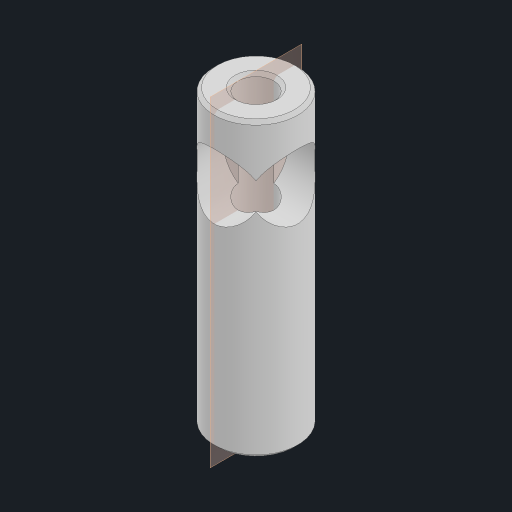
# Autodesk Inventor part: motor_shaft_adapter
Saved by Autodesk Inventor 2023 (Build 270158000, 158)
## iProperties
Created: 2024-04-12
Part Number: motor_shaft_adapter
Material: Generic
Document SubType Name: Modeling
Designer: szymo
Density: 1 g/cm^3
Appearance: Default
Author: szymo
Autodesk Inventor part; units mm, degrees
ref_plane "XZ Plane" through (0, 0, 0) normal (0, 1, 0) x (-1, 0, 0)
ref_plane "XY Plane" through (0, 0, 0) normal (0, 0, 1) x (1, 0, 0)
sketch "Sketch1" plane through (0, 0, 0) normal (0, 1, 0) x (-1, 0, 0)
  circle A0 centre (0, 0) radius 1.1
  circle A1 centre (0, 0) radius 2.575
  dimension "d0" = 2.2
  dimension "d1" = 5.15
  constraints: 2 centre point, 2 coincident
  measures "d0" diameter of A0
  measures "d1" diameter of A1
extrude "Extrusion1" add sketch "Sketch1" along normal blind 18
sketch "Sketch2" plane through (0, 0, 0) normal (0, 0, 1) x (1, 0, 0)
  line L0 (2.575, 18) -> (-2.575, 18) projected
  line L1 (2.575, 0) -> (-2.575, 0) projected
  line L2 (-2.575, 0) -> (-2.575, 18) projected
  line L3 (-2.575, 16) -> (2.5173, 16)
  line L4 (2.575, 18) -> (-2.575, 18) projected
  line L5 (0, 18) -> (0, 0)
  circle A0 centre (0, 14) radius 2
  dimension "d4" = 2
  dimension "d5" = 4
  constraints: 4 end point, 2 point on line, 1 centre point, 1 horizontal, 1 midpoint, 1 parallel, 1 tangent, 1 vertical
  measures "d4" distance between parallel lines of L0 L3
  measures "d5" diameter of A0
extrude "Extrusion2" cut sketch "Sketch2" along normal blind 12 contours A0 L5 | L5 A0
sketch "Sketch3" plane through (0, 0, 0) normal (1, 0, 0) x (0, 1, 0)
  line L0 (18, -2.575) -> (18, 2.575) projected
  line L1 (0, -2.575) -> (0, 2.575) projected
  line L2 (0, 2.575) -> (18, 2.575) projected
  line L3 (16, 2.575) -> (16, -2.525)
  line L4 (18, 1.1) -> (18, -1.1) projected
  line L5 (18, 0) -> (0, 0)
  circle A0 centre (14, 0) radius 2
  point P0 (14, 1.6219)
  dimension "d8" = 2
  dimension "d9" = 4
  constraints: 4 end point, 2 point on line, 1 centre point, 1 horizontal, 1 midpoint, 1 parallel, 1 perpendicular, 1 tangent
  measures "d8" distance between parallel lines of L0 L3
  measures "d9" diameter of A0
extrude "Extrusion3" cut sketch "Sketch3" along normal up to next contours A0 L5 | L5 A0
chamfer "Chamfer1" distance 0.2 angle 45 4 edges at (1.1, 0, 0) (2.575, 0, 0) (1.1, 18, 0) (2.575, 18, 0)
body "Solid1"
